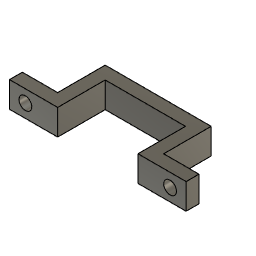
usb-hub-bracket (Autodesk Fusion 360 design; units mm, degrees)
Autodesk Fusion 360 part; units mm, degrees
sketch "Sketch1" plane through (0, 0, 0) normal (0, 0, 1) x (1, 0, 0)
  line L0 (-27.5, 0) -> (-12.5, 0)
  line L1 (-12.5, 0) -> (-12.5, 14.8)
  line L2 (-12.5, 14.8) -> (0, 14.8)
  line L3 (0, 31) -> (0, -29)
  line L4 (27.5, 0) -> (12.5, 0)
  line L5 (12.5, 0) -> (12.5, 14.8)
  line L6 (12.5, 14.8) -> (0, 14.8)
  line L7 (-27.5, 4) -> (-16.5, 4)
  line L8 (-16.5, 4) -> (-16.5, 18.8)
  line L9 (-16.5, 18.8) -> (0, 18.8)
  line L10 (16.5, 18.8) -> (0, 18.8)
  line L11 (16.5, 4) -> (16.5, 18.8)
  line L12 (27.5, 4) -> (16.5, 4)
  line L13 (27.5, 4) -> (27.5, 0)
  line L14 (-27.5, 4) -> (-27.5, 0)
  dimension "d2" = 4
  dimension "d3" = 15
  dimension "d4" = 25
  dimension "d5" = 14.8
  constraint horizontal L0
  constraint perpendicular L0 L1
  constraint perpendicular L1 L2
  constraint vertical L3
  constraint symmetric L0.start L3 L4.start
  constraint symmetric L0.end L3 L4.end
  constraint symmetric L1.end L3 L5.end
  constraint symmetric L2.end L3 L6.end
  constraint perpendicular L4 L13
  constraint perpendicular L0 L14
  measures "d3" distance of L0.start L0.end
  measures "d5" distance of L0.end L2
extrude "Extrude1" add sketch "Sketch1" along normal blind 8
hole "Hole1" at (22.4998, 0, 3.8936) direction (0, 1, 0) diameter 4 depth 5 tip angle 118
hole "Hole2" at (-22.5548, 0, 4.1194) direction (0, 1, 0) diameter 4 depth 5 tip angle 118
